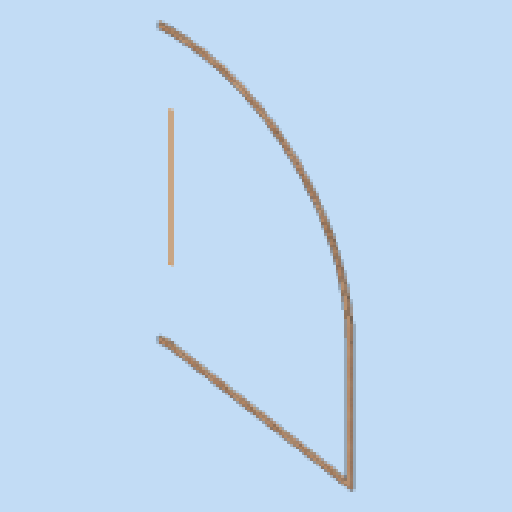
# Autodesk Inventor part: SideWoodL
Saved by Autodesk Inventor 2023 (Build 270158000, 158)
## iProperties
Created: 2026-03-20
Part Number: SideWoodL
Material: Wood (Birch)
Document SubType Name: Modeling
Designer: Nathann
Density: 0.55 g/cm^3
Appearance: Birch - Natural Polished
Author: Nathann
Autodesk Inventor part; units mm, degrees
ref_plane "YZ Plane" through (0, 0, 0) normal (1, 0, 0) x (0, 1, 0)
ref_plane "XZ Plane" through (0, 0, 0) normal (0, 1, 0) x (-1, 0, 0)
ref_plane "XY Plane" through (0, 0, 0) normal (0, 0, 1) x (1, 0, 0)
ref_plane "Work Plane1" through (-210.1828, -2684.477, 12081.7565) normal (0, 0, 1) x (0, -1, 0)
sketch "Sketch3" plane through (-210.1828, -2684.477, 12081.7565) normal (0, 0, 1) x (0, -1, 0)
  line L0 (-680, -79.5954) -> (-730, -79.5954)
  line L1 (-730, -79.5954) -> (-730, 26.2593)
  line L2 (-730, 26.2593) -> (-680, 26.2593)
  line L3 (-680, 26.2593) -> (-680, -79.5954)
  line L4 (1820, -80.7407) -> (1870, -80.7407)
  line L5 (1870, -80.7407) -> (1870, 26.2593)
  line L6 (1870, 26.2593) -> (1820, 26.2593)
  line L7 (1820, 26.2593) -> (1820, -80.7407)
  line L8 (-680, 26.2593) -> (1820, 26.2593)
  arc A0 (970, 1726.2593) -> (-730, 26.2593) centre (970, 26.2593) ccw
  line L9 (970, 26.2593) -> (970, 1726.2593) construction
  line L10 (970, 26.2593) -> (-730, 26.2593) construction
  arc A1 (970, 1676.2593) -> (-680, 26.2593) centre (970, 26.2593) ccw
  line L11 (970, 1676.2593) -> (2111.1765, 1676.2593)
  line L12 (2111.1765, 1676.2593) -> (1820, 26.2593)
  line L13 (1870, 26.2593) -> (2170, 1726.2593)
  line L14 (2170, 1726.2593) -> (970, 1726.2593)
  line L15 (1870, 26.2593) -> (1820, -80.7407)
  point P0 (-2684.477, 210.1828)
  dimension "d18" = 50
  dimension "d19" = 50
  dimension "d20" = 90
  dimension "d21" = 1700
  dimension "d22" = 107
  dimension "d23" = 300
  constraints: 32 end point, 5 parallel, 4 horizontal, 4 point on circle, 2 centre point, 2 coincident, 2 perpendicular, 2 point on line, 1 tangent, 2 other
  measures "d18" distance of L1.end L2.end
  measures "d19" distance of L4.start L4.end
  measures "d20" angle of L9 L10
  measures "d21" radius of A0
  measures "d22" distance of L4.end L5.end
  measures "d23" horizontal distance of L13.end L4.end
extrude "Extrusion1" add sketch "Sketch3" along normal blind 18 contours L0 L1 L2 L3 | L2 A0 L14 L13 L6 L12 L11 A1 | L6 L15 L7
body "Solid1"
